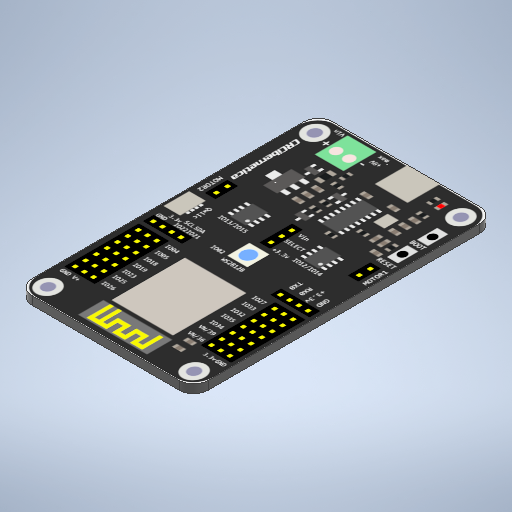
# Autodesk Inventor part: ideaboard
Saved by Autodesk Inventor 2025.2 (Build 292293000, 293)
## iProperties
Created: 2025-06-04
Part Number: ideaboard
Material: Generic
Document SubType Name: Modeling
Designer: cdavi
Density: 1 g/cm^3
Appearance: Default
Finish3_Appearance: Smooth - Black
Finish3_Process: Prime/Paint RAL 3018
Finish3_Description: Prime/Paint RAL 3018
Finish3_ShortDescription: RAL 3018
Finish3_Thickness: 0,050 mm
Finish3_Area: 130,400 mm^2
Author: cdavi
Autodesk Inventor part; units mm, degrees
ref_plane "YZ Plane" through (0, 0, 0) normal (1, 0, 0) x (0, 1, 0)
ref_plane "XZ Plane" through (0, 0, 0) normal (0, 1, 0) x (-1, 0, 0)
ref_plane "XY Plane" through (0, 0, 0) normal (0, 0, 1) x (1, 0, 0)
sketch "Sketch1" plane through (0, 0, 0) normal (0, 1, 0) x (-1, 0, 0)
  line L0 (-21.15, 36.1) -> (-21.15, -36.1)
  line L1 (-21.15, -36.1) -> (21.15, -36.1)
  line L2 (21.15, -36.1) -> (21.15, 36.1)
  line L3 (21.15, 36.1) -> (-21.15, 36.1)
  line L4 (-21.15, 36.1) -> (21.15, -36.1) construction
  line L5 (-21.15, -36.1) -> (21.15, 36.1) construction
  point P0 (0, 0)
  dimension "d0" = 72.2
  dimension "d1" = 42.3
  constraints: 12 end point, 2 midpoint, 2 parallel, 1 perpendicular, 1 vertical
  measures "d0" distance of L1.end L2.end
  measures "d1" distance of L2.end L0.start
extrude "Extrusion1" add sketch "Sketch1" along normal blind 2
sketch "Sketch3" plane through (0, 2, 0) normal (0, 1, 0) x (1, 0, 0)
  line L0 (-21.15, 36.1) -> (-21.15, -36.1) projected
  line L1 (-21.15, 36.1) -> (21.1547, 36.1) construction
  line L2 (21.1547, 36.1) -> (21.1547, -36.1) construction
  line L3 (21.1547, -36.1) -> (-21.15, -36.1) construction
  line L4 (-21.15, -36.1) -> (-21.15, 36.1) construction
  line L5 (21.15, -36.1) -> (21.15, 36.1) projected
  point P0 (0, 0)
  constraints: 1 parallel, 1 vertical, 2 other
sketch "Sketch4" plane through (0, 2, 0) normal (0, 1, 0) x (1, 0, 0)
  line L0 (-21.15, 36.1) -> (-21.15, -36.1) projected
  line L1 (-21.15, -36.1) -> (21.15, -36.1) projected
  line L2 (21.15, -36.1) -> (21.15, 36.1) projected
  line L3 (21.15, 36.1) -> (-21.15, 36.1) projected
  point P0 (0, 0)
fillet "Fillet1" radius 3.5 4 edges at (21.15, 1, 36.1) (-21.15, 1, 36.1) (21.15, 1, -36.1) (-21.15, 1, -36.1)
decal "Decal1"
body "Solid1"
